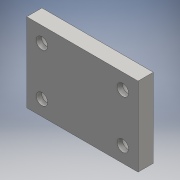
# Autodesk Inventor part: NEMA14 Mounting Bracket
Saved by Autodesk Inventor 2016 (Build 200138000, 138)
## iProperties
Created: 2017-03-15
Part Number: NEMA14 Mounting Bracket
Material: Generic
Document SubType Name: Modeling
Designer: Billy
Density: 1 g/cm^3
Appearance: Default
Author: Billy
Autodesk Inventor part; units mm, degrees
ref_plane "YZ Plane" through (0, 0, 0) normal (1, 0, 0) x (0, 1, 0)
ref_plane "XZ Plane" through (0, 0, 0) normal (0, 1, 0) x (-1, 0, 0)
ref_plane "XY Plane" through (0, 0, 0) normal (0, 0, 1) x (1, 0, 0)
sketch "Sketch1" plane through (0, 0, 0) normal (0, 1, 0) x (-1, 0, 0)
  circle A0 centre (15.9, 35) radius 2.25
  circle A1 centre (15.9, 16) radius 2.25
  circle A2 centre (-15.9, 16) radius 2.25
  circle A3 centre (-15.9, 35) radius 2.25
  line L0 (21.9, 10) -> (-21.9, 10)
  line L1 (-21.9, 10) -> (-21.9, 41)
  line L2 (-21.9, 41) -> (21.9, 41)
  line L3 (21.9, 41) -> (21.9, 10)
  point P0 (0, 0)
  point P1 (0, 0)
  dimension "d0" = 43.8
  dimension "d1" = 31
  constraints: 8 end point, 4 centre point, 2 parallel, 1 horizontal, 1 perpendicular
  measures "d0" distance of L1.end L2.end
  measures "d1" distance of L0.end L1.end
extrude "Extrusion1" add sketch "Sketch1" along normal blind 6
sketch "Sketch2" plane through (0, 6, 0) normal (0, 1, 0) x (1, 0, 0)
  circle A0 centre (-15.9, -16) radius 2.25 projected
  circle A1 centre (-15.9, -16) radius 4
  circle A2 centre (-15.9, -35) radius 2.25 projected
  circle A3 centre (-15.9, -35) radius 4
  circle A4 centre (15.9, -35) radius 2.25 projected
  circle A5 centre (15.9, -35) radius 4
  circle A6 centre (15.9, -16) radius 2.25 projected
  circle A7 centre (15.9, -16) radius 4
  point P0 (0, 0)
  dimension "d4" = 8
  dimension "d5" = 8
  dimension "d6" = 8
  dimension "d7" = 8
  constraints: 4 centre point, 4 coincident
  measures "d4" diameter of A1
  measures "d5" diameter of A3
  measures "d6" diameter of A5
  measures "d7" diameter of A7
extrude "Extrusion2" cut sketch "Sketch2" against normal blind 4
body "Solid1"
